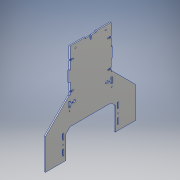
# Autodesk Inventor part: Hopper Wall
Saved by Autodesk Inventor 2018 (Build 220112000, 112)
## iProperties
Created: 2013-10-08
Part Number: Hopper Wall
Material: Aluminum 6061
Document SubType Name: Modeling
Designer: Gabriel Smolnycki
Mass: 680.807 g
Surface Area: 1343.67 cm^2
Volume: 252.151 cm^3
Density: 2.7 g/cm^3
Appearance: Aluminum - Flat
Sending System: SolidWorks 2017
Last Author: Gabriel Smolnycki
Last Saved: 2017-09-14
Author: Gabriel Smolnycki
Autodesk Inventor part; units mm, degrees
ref_plane "XZ Plane" through (0, 0, 0) normal (0, 1, 0) x (-1, 0, 0)
ref_plane "XY Plane" through (0, 0, 0) normal (0, 0, 1) x (1, 0, 0)
ref_plane "Work Plane1" through (-4, 0, 0) normal (1, 0, 0) x (0, 1, 0)
sketch "Sketch1" plane through (-4, 0, 0) normal (1, 0, 0) x (0, 1, 0)
  line L0 (-143.25, -75) -> (-114, -75)
  line L1 (-264.5, -97.85) -> (-285, -97.85)
  line L2 (-47.75, -72) -> (-46.75, -72)
  line L3 (-146.75, -72) -> (-146.75, -75)
  line L4 (-146.75, 72) -> (-147.75, 72)
  line L5 (-47.75, 72) -> (-47.75, 68)
  line L6 (-11, 1.75) -> (-16, 1.75)
  arc A0 (-185.9063, 63.121) -> (-179.834, 64.5065) centre (-182, 60) ccw
  line L7 (-285, -97.85) -> (-285, -102.15)
  line L8 (-173.5, 74.75) -> (-173.5, 79.25)
  line L9 (-46.75, -72) -> (-46.75, -75)
  line L10 (-155.5, -75) -> (-146.75, -75)
  line L11 (-147.75, 72) -> (-147.75, 68)
  line L12 (-47.75, 68) -> (-46.75, 68)
  line L13 (-16, 1.75) -> (-16, -1.75)
  line L14 (-173.5, 79.25) -> (-195, 79.25)
  line L15 (-314.5, -97.85) -> (-335, -97.85)
  line L16 (-76, -75) -> (-46.75, -75)
  line L17 (-155.5, -79) -> (-155.5, -75)
  line L18 (-147.75, 68) -> (-146.75, 68)
  line L19 (-46.75, 68) -> (-46.75, 63)
  line L20 (-16, -1.75) -> (-11, -1.75)
  line L21 (0, 75) -> (-43.25, 75)
  line L22 (-195, 79.25) -> (-195, 74.75)
  line L23 (-335, -97.85) -> (-335, -102.15)
  line L24 (-76, -79) -> (-76, -75)
  line L25 (-241.5, -165) -> (-155.5, -79)
  line L26 (-146.75, 68) -> (-146.75, 63)
  line L27 (-46.75, 63) -> (-43.25, 63)
  line L28 (-11, -1.75) -> (-11, -2.75)
  line L29 (-195, 74.75) -> (-191.5, 74.75)
  line L30 (-335, -102.15) -> (-314.5, -102.15)
  line L31 (-114, -79) -> (-76, -79)
  line L32 (-355, -165) -> (-241.5, -165)
  line L33 (-146.75, 63) -> (-143.25, 63)
  line L34 (-43.25, 63) -> (-43.25, 68)
  line L35 (-11, -2.75) -> (-7, -2.75)
  line L36 (-114, -75) -> (-114, -79)
  line L37 (-355, -90) -> (-355, -165)
  line L38 (-143.25, 63) -> (-143.25, 68)
  line L39 (-43.25, 68) -> (-42.25, 68)
  line L40 (-7, -2.75) -> (-7, -1.75)
  line L41 (-314.5, -102.15) -> (-314.5, -97.85)
  line L42 (0, -75) -> (0, -20)
  line L43 (-270, -90) -> (-355, -90)
  line L44 (-143.25, 68) -> (-142.25, 68)
  line L45 (-42.25, 68) -> (-42.25, 72)
  line L46 (-7, -1.75) -> (-4, -1.75)
  line L47 (-335, 102.15) -> (-335, 97.85)
  line L48 (-43.25, -75) -> (0, -75)
  line L49 (-143.25, -75) -> (-143.25, -72)
  line L50 (-255, -75) -> (-270, -90)
  line L51 (-142.25, 68) -> (-142.25, 72)
  line L52 (-42.25, 72) -> (-43.25, 72)
  line L53 (-4, -1.75) -> (-4, -20)
  arc A1 (-179.834, -64.5065) -> (-185.9063, -63.121) centre (-182, -60) ccw
  line L54 (-195, -74.75) -> (-195, -79.25)
  line L55 (-335, 97.85) -> (-314.5, 97.85)
  line L56 (-43.25, -75) -> (-43.25, -72)
  line L57 (-143.25, -72) -> (-142.25, -72)
  line L58 (-255, 75) -> (-255, -75)
  line L59 (-142.25, 72) -> (-143.25, 72)
  line L60 (-43.25, 72) -> (-43.25, 75)
  line L61 (-4, -20) -> (0, -20)
  arc A2 (-191.5, -74.75) -> (-185.9063, -63.121) centre (-191.5, -67.5902) ccw
  line L62 (-46.75, 75) -> (-76, 75)
  line L63 (-195, -79.25) -> (-173.5, -79.25)
  line L64 (-314.5, 97.85) -> (-314.5, 102.15)
  line L65 (-43.25, -72) -> (-42.25, -72)
  line L66 (-142.25, -72) -> (-142.25, -68)
  line L67 (-270, 90) -> (-255, 75)
  line L68 (-143.25, 72) -> (-143.25, 75)
  line L69 (-191.5, -74.75) -> (-195, -74.75)
  line L70 (-146.75, 75) -> (-155.5, 75)
  line L71 (-173.5, -79.25) -> (-173.5, -74.75)
  line L72 (-42.25, -72) -> (-42.25, -68)
  line L73 (-142.25, -68) -> (-143.25, -68)
  line L74 (-355, 90) -> (-270, 90)
  line L75 (-114, 75) -> (-143.25, 75)
  line L76 (0, 20) -> (0, 75)
  line L77 (-314.5, 102.15) -> (-335, 102.15)
  line L78 (-177.5, 74.75) -> (-173.5, 74.75)
  line L79 (-173.5, -74.75) -> (-177.5, -74.75)
  line L80 (-285, 102.15) -> (-285, 97.85)
  line L81 (-42.25, -68) -> (-43.25, -68)
  line L82 (-143.25, -68) -> (-143.25, -63)
  line L83 (-355, 165) -> (-355, 90)
  line L84 (-114, 79) -> (-114, 75)
  line L85 (0, 20) -> (-4, 20)
  arc A3 (-179.834, -64.5065) -> (-177.5, -74.75) centre (-177.5, -69.3623) ccw
  line L86 (-285, 97.85) -> (-264.5, 97.85)
  line L87 (-43.25, -68) -> (-43.25, -63)
  line L88 (-143.25, -63) -> (-146.75, -63)
  line L89 (-241.5, 165) -> (-355, 165)
  line L90 (-76, 79) -> (-114, 79)
  line L91 (-4, 20) -> (-4, 1.75)
  line L92 (-264.5, 97.85) -> (-264.5, 102.15)
  line L93 (-43.25, -63) -> (-46.75, -63)
  line L94 (-146.75, -63) -> (-146.75, -68)
  line L95 (-155.5, 79) -> (-241.5, 165)
  line L96 (-76, 75) -> (-76, 79)
  line L97 (-4, 1.75) -> (-7, 1.75)
  line L98 (-264.5, 102.15) -> (-285, 102.15)
  line L99 (-46.75, -63) -> (-46.75, -68)
  line L100 (-146.75, -68) -> (-147.75, -68)
  line L101 (-155.5, 75) -> (-155.5, 79)
  line L102 (-7, 1.75) -> (-7, 2.75)
  line L103 (-285, -102.15) -> (-264.5, -102.15)
  line L104 (-46.75, -68) -> (-47.75, -68)
  line L105 (-147.75, -68) -> (-147.75, -72)
  line L106 (-46.75, 75) -> (-46.75, 72)
  line L107 (-7, 2.75) -> (-11, 2.75)
  arc A4 (-185.9063, 63.121) -> (-191.5, 74.75) centre (-191.5, 67.5902) ccw
  arc A5 (-177.5, 74.75) -> (-179.834, 64.5065) centre (-177.5, 69.3623) ccw
  line L108 (-264.5, -102.15) -> (-264.5, -97.85)
  line L109 (-47.75, -68) -> (-47.75, -72)
  line L110 (-147.75, -72) -> (-146.75, -72)
  line L111 (-146.75, 75) -> (-146.75, 72)
  line L112 (-46.75, 72) -> (-47.75, 72)
  line L113 (-11, 2.75) -> (-11, 1.75)
  constraints: 228 end point, 74 equal length, 56 horizontal, 54 vertical, 17 collinear, 12 point on circle, 6 centre point, 1 equal radius, 1 parallel, 1 perpendicular
extrude "Extrusion1" add sketch "Sketch1" along normal blind 4.064
hole "Hole6" at (-4, -299.75, -100) direction (1, 0, 0) diameter 3.5 depth 4.064 tip angle 118
hole "Hole5" at (-4, -299.75, 100) direction (1, 0, 0) diameter 3.5 depth 4.064 tip angle 118
hole "Hole4" at (-4, -205, -77) direction (1, 0, 0) diameter 3.5 depth 4.064 tip angle 118
sketch "Sketch4" plane through (-4, 0, 0) normal (1, 0, 0) x (0, 1, 0)
  point P0 (-205, -77)
hole "Hole3" at (-4, -205, 77) direction (1, 0, 0) diameter 3.5 depth 4.064 tip angle 118
sketch "Sketch3" plane through (-4, 0, 0) normal (1, 0, 0) x (0, 1, 0)
  point P0 (-299.75, 100)
hole "Hole2" at (-4, -14.5, 55) direction (1, 0, 0) diameter 4.5 depth 4.064 tip angle 118
sketch "Sketch2" plane through (-4, 0, 0) normal (1, 0, 0) x (0, 1, 0)
  point P0 (-299.75, -100)
hole "Hole1" at (-4, -14.5, -55) direction (1, 0, 0) diameter 4.5 depth 4.064 tip angle 118
sketch "Sketch5" plane through (-4, 0, 0) normal (1, 0, 0) x (0, 1, 0)
  point P0 (-205, 77)
sketch "Sketch6" plane through (-4, 0, 0) normal (1, 0, 0) x (0, 1, 0)
  point P0 (-14.5, 55)
sketch "Sketch7" plane through (-4, 0, 0) normal (1, 0, 0) x (0, 1, 0)
  point P0 (-14.5, -55)
body "Solid3"
